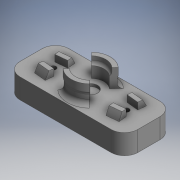
# Autodesk Inventor part: MG996R Arm Test
Saved by Autodesk Inventor 2020.5 (Build 245400000, 400)
## iProperties
Created: 2023-03-16
Part Number: MG996R Arm Test
Material: Generic
Document SubType Name: Modeling
Designer: Wes
Density: 1 g/cm^3
Appearance: Default
Author: Wes
Autodesk Inventor part; units mm, degrees
ref_plane "YZ Plane" through (0, 0, 0) normal (1, 0, 0) x (0, 1, 0)
ref_plane "XZ Plane" through (0, 0, 0) normal (0, 1, 0) x (-1, 0, 0)
ref_plane "XY Plane" through (0, 0, 0) normal (0, 0, 1) x (1, 0, 0)
sketch "Base" plane through (0, 0, 0) normal (0, 0, 1) x (1, 0, 0)
  line L0 (0, 0) -> (-22, 0)
  line L1 (-22, 0) -> (-22, 53)
  line L2 (-22, 53) -> (0, 53)
  line L3 (0, 53) -> (0, 0)
  line L4 (-11, 26.5) -> (-11, 43.6) construction
  line L5 (-11, 26.5) -> (-11, 9.4) construction
  line L6 (-11, 26.5) -> (-11, 10.7) construction
  line L7 (-11, 26.5) -> (-11, 42.3) construction
  line L8 (-11, 10.7) -> (-11, 9.4) construction
  line L9 (-11, 42.3) -> (-11, 43.6) construction
  circle A0 centre (-11, 42.95) radius 1.175
  circle A1 centre (-11, 10.05) radius 1.175
  dimension "d0" = 22
  dimension "d1" = 53
  dimension "d8" = 34.2
  dimension "d14" = 31.6
  dimension "d15" = 2.35
  dimension "d16" = 2.35
  constraints: 20 end point, 3 vertical, 2 centre point, 2 midpoint, 2 parallel, 2 point on line, 1 collinear, 1 horizontal, 1 perpendicular
  measures "d0" distance of L1.end L2.end
  measures "d1" distance of L0.end L1.end
  measures "d8" distance of L4.end L5.end
  measures "d14" distance of L7.end L6.end
  measures "d15" diameter of A0
  measures "d16" diameter of A1
extrude "Extrusion1" add sketch "Base" along normal mid plane 9
sketch "Countersink Arm Screw Holes" plane through (0, 0, -4.5) normal (0, 0, -1) x (-1, 0, 0)
  circle A0 centre (11, 10.05) radius 1.175 projected
  circle A1 centre (11, 10.05) radius 2.7
  circle A2 centre (11, 42.95) radius 1.175 projected
  circle A3 centre (11, 42.95) radius 2.7
  point P0 (0, 0)
  dimension "d19" = 5.4
  dimension "d20" = 5.4
  constraints: 2 centre point, 2 coincident
  measures "d19" diameter of A1
  measures "d20" diameter of A3
extrude "Extrusion2" cut sketch "Countersink Arm Screw Holes" against normal blind 1.5 contours A0 | A1 | A2 | A3
sketch "Axle Screw Countersink" plane through (0, 0, 4.5) normal (0, 0, 1) x (1, 0, 0)
  circle A0 centre (-11.089431, 26.715447) radius 3.1
  point P0 (0, 0)
  dimension "d23" = 6.2
  constraints: 1 centre point
  measures "d23" diameter of A0
extrude "Extrusion3" cut sketch "Axle Screw Countersink" against normal blind 1.2
sketch "Arm Center Fitting" plane through (0, 0, 4.5) normal (0, 0, 1) x (1, 0, 0)
  circle A0 centre (-11.089431, 26.715447) radius 5.975 construction
  line L0 (-6.696468, 22.665447) -> (-6.696468, 30.765447) construction
  line L1 (-6.696468, 22.665447) -> (-15.482394, 22.665447) construction
  line L2 (-15.482394, 22.665447) -> (-15.482394, 30.765447) construction
  arc A1 (-15.482394, 30.765447) -> (-15.482394, 22.665447) centre (-11.089431, 26.715447) ccw
  line L3 (-15.482394, 22.665447) -> (-17.320454, 20.970886)
  line L4 (-15.482394, 30.765447) -> (-17.320454, 32.460008)
  arc A2 (-17.320454, 32.460008) -> (-17.320454, 20.970886) centre (-11.089431, 26.715447) ccw
  line L5 (-11.089431, 16.056342) -> (-11.089431, 38.404771) construction
  arc A3 (-6.696468, 22.665447) -> (-6.696468, 30.765447) centre (-11.089431, 26.715447) ccw
  line L6 (-6.696468, 22.665447) -> (-4.858408, 20.970886)
  line L7 (-6.696468, 30.765447) -> (-4.858408, 32.460008)
  arc A4 (-4.858408, 20.970886) -> (-4.858408, 32.460008) centre (-11.089431, 26.715447) ccw
  point P0 (0, 0)
  dimension "d27" = 11.95
  dimension "d31" = 8.1
  dimension "d32" = 8.1
  dimension "d33" = 2.5
  dimension "d34" = 2.5
  constraints: 16 end point, 12 point on circle, 5 centre point, 2 line through centre, 2 symmetric about line, 2 vertical, 1 coincident, 1 concentric, 1 perpendicular, 2 other
  measures "d27" diameter of A0
  measures "d31" distance of L0.start L0.end
  measures "d32" distance of L1.end L2.end
  measures "d33" distance of L1.end L3.end
  measures "d34" distance of L2.end L4.end
extrude "Extrusion4" add sketch "Arm Center Fitting" along normal blind 5
sketch "Rotation Support" plane through (0, 0, 9.5) normal (0, 0, 1) x (1, 0, 0)
  line L0 (-17.064431, 26.715447) -> (-17.864431, 26.715447) construction
  circle A0 centre (-11.089431, 26.715447) radius 6.775 construction
  arc A1 (-16.070573, 31.307707) -> (-16.070573, 22.123188) centre (-11.089431, 26.715447) ccw
  line L1 (-17.864431, 26.715447) -> (-19.864431, 26.715447) construction
  circle A2 centre (-11.089431, 26.715447) radius 8.775 construction
  arc A3 (-17.541021, 32.663355) -> (-17.541021, 20.767539) centre (-11.089431, 26.715447) ccw
  line L2 (-17.541021, 20.767539) -> (-16.070573, 22.123188)
  line L3 (-15.482394, 22.665447) -> (-17.320454, 20.970886)
  line L4 (-16.070573, 31.307707) -> (-17.541021, 32.663355)
  line L5 (-17.320454, 32.460008) -> (-15.482394, 30.765447)
  line L6 (-11.089431, 15.244922) -> (-11.089431, 38.763368) construction
  arc A4 (-6.108289, 22.123188) -> (-6.108289, 31.307707) centre (-11.089431, 26.715447) ccw
  arc A5 (-4.637841, 20.767539) -> (-4.637841, 32.663355) centre (-11.089431, 26.715447) ccw
  line L7 (-4.637841, 20.767539) -> (-6.108289, 22.123188)
  line L8 (-6.108289, 31.307707) -> (-4.637841, 32.663355)
  point P0 (0, 0)
  dimension "d38" = 0.8
  dimension "d39" = 2
  constraints: 16 point on circle, 14 end point, 6 centre point, 4 symmetric about line, 2 coincident, 2 collinear, 2 horizontal, 1 concentric, 1 vertical, 2 other
  measures "d38" distance of L0.start L0.end
  measures "d39" distance of L0.end L1.end
extrude "Extrusion5" add sketch "Rotation Support" along normal blind 3.25
sketch "Arm Support" plane through (0, 0, 4.5) normal (0, 0, 1) x (1, 0, 0)
  circle A0 centre (-11, 10.05) radius 1.175 construction
  line L0 (-11, 8.875) -> (-11, 13.375) construction
  line L1 (-11, 13.375) -> (-7.875, 13.375) construction
  line L2 (-11, 13.375) -> (-14.125, 13.375) construction
  line L3 (-17.064431, 26.715447) -> (-5.114431, 26.715447) construction
  line L4 (-11, 10.05) -> (-8.2, 10.05) construction
  line L5 (-11, 10.05) -> (-8.2, 10.05) construction
  line L6 (-11, 10.05) -> (-13.8, 10.05) construction
  line L7 (-11, 10.05) -> (-8.2, 10.05) construction
  line L8 (-14.125, 13.375) -> (-13.8, 10.05)
  line L9 (-13.8, 10.05) -> (-15.790514, 9.855438)
  line L10 (-15.790514, 9.855438) -> (-16.115514, 13.180438)
  line L11 (-16.115514, 13.180438) -> (-14.125, 13.375)
  line L12 (-7.875, 13.375) -> (-8.2, 10.05)
  line L13 (-8.2, 10.05) -> (-6.209486, 9.855438)
  line L14 (-6.209486, 9.855438) -> (-5.884486, 13.180438)
  line L15 (-5.884486, 13.180438) -> (-7.875, 13.375)
  line L16 (-13.8, 10.05) -> (-13.605438, 8.059486)
  line L17 (-13.605438, 8.059486) -> (-15.595952, 7.864925)
  line L18 (-15.595952, 7.864925) -> (-15.790514, 9.855438)
  line L19 (-8.2, 10.05) -> (-8.394562, 8.059486)
  line L20 (-8.394562, 8.059486) -> (-6.404048, 7.864925)
  line L21 (-6.404048, 7.864925) -> (-6.209486, 9.855438)
  line L22 (-14.125, 40.055894) -> (-13.8, 43.380894)
  line L23 (-13.8, 43.380894) -> (-15.790514, 43.575456)
  line L24 (-15.790514, 43.575456) -> (-16.115514, 40.250456)
  line L25 (-16.115514, 40.250456) -> (-14.125, 40.055894)
  line L26 (-7.875, 40.055894) -> (-8.2, 43.380894)
  line L27 (-8.2, 43.380894) -> (-6.209486, 43.575456)
  line L28 (-5.884486, 40.250456) -> (-7.875, 40.055894)
  line L29 (-6.209486, 43.575456) -> (-5.884486, 40.250456)
  line L30 (-13.8, 43.380894) -> (-13.605438, 45.371408)
  line L31 (-13.605438, 45.371408) -> (-15.595952, 45.56597)
  line L32 (-15.595952, 45.56597) -> (-15.790514, 43.575456)
  line L33 (-8.2, 43.380894) -> (-8.394562, 45.371408)
  line L34 (-8.394562, 45.371408) -> (-6.404048, 45.56597)
  line L35 (-6.404048, 45.56597) -> (-6.209486, 43.575456)
  point P0 (0, 0)
  dimension "d45" = 4.5
  dimension "d51" = 6.25
  dimension "d63" = 5.6
  dimension "d64" = 2
  dimension "d65" = 2
  constraints: 72 end point, 18 symmetric about line, 7 horizontal, 5 perpendicular, 2 collinear, 1 vertical, 1 vertical alignment, 1 other
  measures "d45" distance of L0.start L0.end
  measures "d51" distance of L2.end L1.end
  measures "d63" distance of L6.end L4.end
  measures "d64" distance of L6.end L9.end
  measures "d65" distance of L6.end L16.end
extrude "Extrusion6" add sketch "Arm Support" along normal blind 3
draft "FaceDraft1" angle 28 pull direction (0, 0, 1) faces at (-6.23086, 9.636763, 5.5) (-6.057673, 42.022294, 5.5) fixed edges at (-6.144267, 10.522682, 7.5) (-6.144267, 42.908213, 7.5)
draft "FaceDraft2" angle 28 pull direction (0, 0, 1) faces at (-15.942327, 11.4086, 5.5) (-15.76914, 43.794132, 5.5) fixed edges at (-15.855733, 10.522682, 7.5) (-15.855733, 42.908213, 7.5)
fillet "Fillet1" radius 2 6 edges at (-17.8644, 26.7154, 9.5) (-4.3144, 26.7154, 9.5) (-19.5644, 26.7154, 4.5) (-2.6144, 26.7154, 4.5) (-19.5644, 26.7154, 9.5) (-2.6144, 26.7154, 9.5)
fillet "Fillet2" radius 6 4 edges at (0, 0, 0) (0, 53, 0) (-22, 53, 0) (-22, 0, 0)
body "Solid1"
